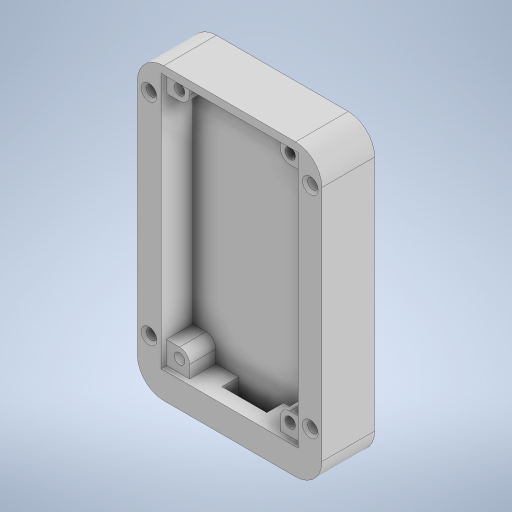
# Autodesk Inventor part: 하우징
Saved by Autodesk Inventor 2023 (Build 270158000, 158)
## iProperties
Created: 2022-06-15
Part Number: 하우징
Material: 일반
Document SubType Name: Modeling
Designer: user
Density: 1 g/cm^3
Appearance: 기본값
Author: user
Autodesk Inventor part; units mm, degrees
ref_plane "YZ Plane" through (0, 0, 0) normal (1, 0, 0) x (0, 1, 0)
ref_plane "XZ Plane" through (0, 0, 0) normal (0, 1, 0) x (-1, 0, 0)
ref_plane "XY Plane" through (0, 0, 0) normal (0, 0, 1) x (1, 0, 0)
sketch "스케치1" plane through (0, 0, 0) normal (0, 0, 1) x (1, 0, 0)
  line L0 (-17.5, 29.25) -> (17.5, 29.25)
  line L1 (17.5, 29.25) -> (17.5, -29.25)
  line L2 (17.5, -29.25) -> (-17.5, -29.25)
  line L3 (-17.5, -29.25) -> (-17.5, 29.25)
  line L4 (-17.5, 29.25) -> (17.5, -29.25) construction
  line L5 (17.5, 29.25) -> (-17.5, -29.25) construction
  line L6 (-13, -24.25) -> (13, -24.25)
  line L7 (13, -24.25) -> (13, 24.25)
  line L8 (13, 24.25) -> (-13, 24.25)
  line L9 (-13, 24.25) -> (-13, -24.25)
  line L10 (-13, -24.25) -> (13, 24.25) construction
  line L11 (13, -24.25) -> (-13, 24.25) construction
  line L12 (-9.5, 24.25) -> (9.5, 24.25)
  line L13 (9.5, 24.25) -> (9.5, -24.25)
  line L14 (9.5, -24.25) -> (-9.5, -24.25)
  line L15 (-9.5, -24.25) -> (-9.5, 24.25)
  line L16 (-9.5, 24.25) -> (9.5, -24.25) construction
  line L17 (9.5, 24.25) -> (-9.5, -24.25) construction
  line L18 (17.5, 25.75) -> (-17.5, 25.75)
  point P0 (0, 0)
  dimension "d0" = 58.5
  dimension "d1" = 35
  dimension "d2" = 26
  dimension "d3" = 48.5
  dimension "d4" = 3.5
  dimension "d10" = 1.5
  constraints: 38 end point, 6 midpoint, 6 parallel, 4 perpendicular, 3 horizontal, 3 point on line
  measures "d0" distance of L2.end L0.start
  measures "d1" distance of L0.start L0.end
  measures "d2" distance of L8.end L7.end
  measures "d3" distance of L7.end L6.end
  measures "d4" distance between parallel lines of L7 L13
  measures "d10" distance between parallel lines of L12 L18
extrude "돌출1" add sketch "스케치1" against normal blind 10 contours L18 L1 L2 L3 | L9 L8 L15 L6 | L15 L8 L13 L6 | L13 L8 L7 L6
extrude "돌출3" cut sketch "스케치1" against normal blind 6 contours L9 L8 L15 L6 | L15 L8 L13 L6 | L13 L8 L7 L6
sketch "스케치2" plane through (0, 0, -6) normal (0, 0, 1) x (1, 0, 0)
  circle A0 centre (10.5, 22.35) radius 1
  line L0 (10.5, 22.35) -> (-10.5, 22.35) construction
  line L1 (-13, 24.25) -> (13, 24.25) construction
  line L2 (0, 0) -> (0, 7.5455)
  circle A1 centre (-10.5, 22.35) radius 1
  line L3 (-13, 24.25) -> (13, 24.25) projected
  line L4 (0, 24.25) -> (0, -23.75) construction
  line L5 (0, 0.25) -> (5.5908, 0.25)
  circle A2 centre (10.5, -21.85) radius 1
  circle A3 centre (-10.5, -21.85) radius 1
  circle A4 centre (-10.5, 22.35) radius 1.9
  circle A5 centre (10.5, 22.35) radius 1.9
  circle A6 centre (10.5, -21.85) radius 1.9
  circle A7 centre (-10.5, -21.85) radius 1.9
  line L6 (-8.6, -21.85) -> (-8.6, -24.25)
  line L7 (13, -24.25) -> (-13, -24.25) projected
  line L8 (-10.5, -19.95) -> (-13, -19.95)
  line L9 (-13, -24.25) -> (-13, 24.25) projected
  line L10 (13, 24.25) -> (13, -24.25) projected
  line L11 (10.5, -19.95) -> (13, -19.95)
  line L12 (8.6, -21.85) -> (8.6, -24.25)
  line L13 (-8.6, 22.35) -> (-8.6, 24.75)
  line L14 (-10.5, 20.45) -> (-13, 20.45)
  line L15 (10.5, 20.45) -> (13, 20.45)
  line L16 (8.6, 22.35) -> (8.6, 24.75)
  point P0 (0, 22.35)
  point P1 (8.6, 24.25)
  point P2 (-8.6, 24.25)
  dimension "d13" = 2
  dimension "d14" = 21
  dimension "d15" = 1.9
  dimension "d16" = 48
  dimension "d17" = 3.8
  dimension "d18" = 3.8
  constraints: 24 end point, 11 symmetric about line, 8 centre point, 5 coincident, 4 point on circle, 4 point on line, 4 tangent, 3 horizontal, 3 midpoint, 3 vertical, 2 perpendicular, 1 vertical alignment, 3 other
  measures "d13" diameter of A0
  measures "d14" distance of L0.start L0.end
  measures "d15" distance between parallel lines of L1 L0
  measures "d16" distance of L4.start L4.end
  measures "d17" diameter of A6
  measures "d18" diameter of A7
extrude "돌출4" add sketch "스케치2" along normal blind 6 contours L3 A4 L14 L9 | L3 L13 A4 | A4 | L8 A7 L6 L7 L9 | L3 A5 L16 | A7 | L3 L10 L15 A5 | A5 | L12 A6 L11 L10 L7 | A6
sketch "스케치3" plane through (0, 0, 0) normal (0, 0, 1) x (1, 0, 0)
  line L0 (-8.6, 24.25) -> (8.6, 24.25) projected
  line L1 (-8.6, 24.25) -> (-13, 24.25)
  line L2 (-13, 24.25) -> (13, 24.25)
  line L3 (13, 24.25) -> (13, -24.25)
  line L4 (13, -24.25) -> (-13, -24.25)
  line L5 (-13, -24.25) -> (-13, 24.25)
  circle A0 centre (-10.5, -21.85) radius 1 projected
  circle A1 centre (10.5, 22.35) radius 1 projected
  circle A2 centre (10.5, -21.85) radius 1 projected
  circle A3 centre (-10.5, 22.35) radius 1 projected
  line L6 (-13, -19.95) -> (-13, 20.45) projected
  line L7 (-13, 20.45) -> (-10.5, 20.45) projected
  arc A4 (-10.5, 20.45) -> (-8.6, 22.35) centre (-10.5, 22.35) ccw projected
  line L8 (-8.6, 22.35) -> (-8.6, 24.25) projected
  line L9 (-8.6, 24.25) -> (8.6, 24.25) projected
  line L10 (8.6, 24.25) -> (8.6, 22.35) projected
  arc A5 (8.6, 22.35) -> (10.5, 20.45) centre (10.5, 22.35) ccw projected
  line L11 (10.5, 20.45) -> (13, 20.45) projected
  line L12 (13, 20.45) -> (13, -19.95) projected
  line L13 (13, -19.95) -> (10.5, -19.95) projected
  arc A6 (10.5, -19.95) -> (8.6, -21.85) centre (10.5, -21.85) ccw projected
  line L14 (8.6, -21.85) -> (8.6, -24.25) projected
  line L15 (8.6, -24.25) -> (-8.6, -24.25) projected
  line L16 (-8.6, -24.25) -> (-8.6, -21.85) projected
  arc A7 (-8.6, -21.85) -> (-10.5, -19.95) centre (-10.5, -21.85) ccw projected
  line L17 (-10.5, -19.95) -> (-13, -19.95) projected
  line L18 (17.5, -29.25) -> (17.5, 25.75) projected
  line L19 (17.5, 25.75) -> (-17.5, 25.75) projected
  line L20 (-17.5, 25.75) -> (-17.5, -29.25) projected
  line L21 (-17.5, -29.25) -> (17.5, -29.25) projected
  point P0 (0, 0)
  dimension "d21" = 26
  dimension "d22" = 48.5
  constraints: 10 end point, 2 horizontal, 2 parallel, 1 perpendicular
  measures "d21" distance of L3.end L4.end
  measures "d22" distance of L2.end L3.end
extrude "돌출5" cut sketch "스케치3" against normal blind 1 contours L8 A4 L7 L5 L1 | L0 L10 A5 L11 L3 L13 A6 L14 L4 L16 A7 L17 L5 L7 A4 L8 | L2 L3 L11 A5 L10 | L17 A7 L16 L4 L5 | L3 L4 L14 A6 L13 | A0 | A1 | A2 | A3
sketch "스케치4" plane through (-13, -24.25, 0) normal (0, 1, 0) x (1, 0, 0)
  line L0 (8.75, 9.2) -> (17.25, 9.2)
  line L1 (17.25, 9.2) -> (17.25, 2.8)
  line L2 (17.25, 2.8) -> (8.75, 2.8)
  line L3 (8.75, 2.8) -> (8.75, 9.2)
  line L4 (4.4, 6) -> (21.6, 6) projected
  line L5 (8.75, 9.2) -> (17.25, 2.8) construction
  line L6 (17.25, 9.2) -> (8.75, 2.8) construction
  point P0 (13, 0)
  point P1 (13, 6)
  point P2 (17.25, 6)
  point P3 (8.75, 6)
  dimension "d25" = 8.5
  dimension "d26" = 6.4
  constraints: 12 end point, 3 midpoint, 2 parallel, 1 horizontal, 1 perpendicular
  measures "d25" distance of L1.end L2.end
  measures "d26" distance of L2.end L0.start
extrude "돌출6" cut sketch "스케치4" against normal blind 5 contours L4 L1 L2 L3
fillet "모깎기2" radius 5 4 edges at (17.5, -29.25, -5) (-17.5, -29.25, -5) (17.5, 25.75, -5) (-17.5, 25.75, -5)
sketch "스케치5" plane through (0, 0, 0) normal (0, 0, 1) x (1, 0, 0)
  circle A0 centre (15.3, -20) radius 1
  line L0 (0, 0) -> (0, -10.3102)
  circle A1 centre (-15.3, -20) radius 1
  line L1 (0, 0) -> (6.1886, 0)
  circle A2 centre (15.3, 20) radius 1
  circle A3 centre (-15.3, 20) radius 1
  dimension "d30" = 2
  dimension "d31" = 20
  dimension "d32" = 15.3
  constraints: 4 centre point, 4 end point, 3 symmetric about line, 1 horizontal, 1 vertical, 3 other
  measures "d30" diameter of A0
  measures "d31" vertical distance of A0.centre L0.start
  measures "d32" horizontal distance of L0.start A0.centre
extrude "돌출7" cut sketch "스케치5" against normal blind 5
chamfer "모따기1" distance 0.5 angle 45 4 edges at (-16.3, 20, 0) (14.3, 20, 0) (14.3, -20, 0) (-16.3, -20, 0)
